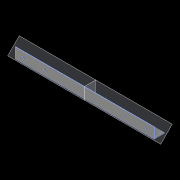
# Autodesk Inventor part: Lbarx1 big
Saved by Autodesk Inventor 2016 (Build 200138000, 138)
## iProperties
Created: 2019-02-12
Part Number: Lbarx1 big
Material: Aluminum 6061
Document SubType Name: Modeling
Designer: Calb3e
Density: 2.7 g/cm^3
Appearance: Aluminum - Flat
Author: Calb3e
Autodesk Inventor part; units mm, degrees
ref_plane "XZ Plane" through (0, 0, 0) normal (0, 1, 0) x (-1, 0, 0)
ref_plane "XY Plane" through (0, 0, 0) normal (0, 0, 1) x (1, 0, 0)
sketch "Sketch1" plane through (0, 0, 0) normal (0, 1, 0) x (-1, 0, 0)
  line L0 (0, 0) -> (-330, 0)
  line L1 (-330, 0) -> (-330, 25)
  line L2 (-330, 25) -> (0, 25)
  line L3 (0, 25) -> (0, 0)
  dimension "d0" = 330
  dimension "d1" = 25
  constraints: 8 end point, 2 parallel, 1 horizontal, 1 perpendicular
  measures "d0" distance of L0.start L0.end
  measures "d1" distance of L2.end L0.start
extrude "Extrusion1" add sketch "Sketch1" along normal blind 1
sketch "Sketch2" plane through (0, 1, 0) normal (0, 1, 0) x (1, 0, 0)
  line L0 (0, 0) -> (330, 0)
  line L1 (330, 0) -> (330, -1)
  line L2 (330, -1) -> (0, -1)
  line L3 (0, -1) -> (0, 0)
  dimension "d4" = 330
  dimension "d5" = 1
  constraints: 8 end point, 2 parallel, 1 horizontal, 1 perpendicular
  measures "d4" distance of L0.start L0.end
  measures "d5" distance of L0.end L1.end
extrude "Extrusion2" add sketch "Sketch2" along normal blind 24
hole "Hole1" at (20, 12.4367, 1) direction (0, 0, -1) diameter 5.5 end through all
pattern_linear "Rectangular Pattern1" count 2 spacing 50 along (1, 0, 0) of "Hole1"
ref_plane "Work Plane1" through (165, 0, 0) normal (1, 0, 0) x (0, 1, 0)
mirror "Mirror1" about plane through (165, 0, 0) normal (1, 0, 0) of "Hole1", "Rectangular Pattern1"
ref_plane "Work Plane2" through (82.5, 1, 1) normal (0, -0.7071, 0.7071) x (-1, 0, 0)
mirror "Mirror2" about plane through (82.5, 1, 1) normal (0, -0.7071, 0.7071) of "Extrusion2", "Hole1", "Rectangular Pattern1", "Mirror1"
body "Solid1"
